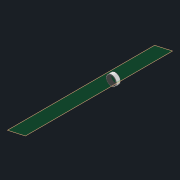
# Autodesk Inventor part: Ball Screw Nut Cap
Saved by Autodesk Inventor 2021 (Build 250183000, 183)
## iProperties
Created: 2020-10-16
Part Number: Ball Screw Nut Cap
Material: Generic
Document SubType Name: Modeling
Designer: Eugene Tang
Density: 1 g/cm^3
Appearance: Default
Mass: 34.4311 g
Surface Area: 123.547 cm^2
Volume: 34.4311 cm^3
Author: Eugene Tang
Autodesk Inventor part; units mm, degrees
ref_plane "YZ Plane" through (0, 0, 0) normal (1, 0, 0) x (0, 1, 0)
ref_plane "XZ Plane" through (0, 0, 0) normal (0, 1, 0) x (-1, 0, 0)
ref_plane "XY Plane" through (0, 0, 0) normal (0, 0, 1) x (1, 0, 0)
sketch "Sketch3" plane through (0, 0, 0) normal (0, 0, 1) x (1, 0, 0)
  circle A0 centre (0.7808, 0) radius 22.0799
  circle A1 centre (0.7808, 0) radius 42.0799
  circle A2 centre (0.7808, 0) radius 18.8799 projected
  dimension "d0" = 44.1598
  dimension "d2" = 20
  constraints: 2 centre point, 1 coincident, 1 concentric
  measures "d0" diameter of A0
  measures "d2" radial gap between concentric circles of A1 A0
extrude "Extrusion1" add sketch "Sketch3" against normal blind 20 contours A1
ref_plane "Work Plane1" through (0.7808, 0, -201) normal (0.2200222, -0.9754949, 0) x (-0.9754949, -0.2200222, 0)
sketch "Sketch5" plane through (0.7808, 0, -201) normal (0.2200222, -0.9754949, 0) x (-0.9754949, -0.2200222, 0)
  line L0 (22.0799, -201) -> (-22.0799, -201) construction
  line L1 (-22.0799, -201) -> (-22.0799, -215.8832) construction
  line L2 (-21.9175, -201) -> (-21.9175, -215.8832) construction
  line L3 (-21.9175, -202.5) -> (-27.3833, -202.5) construction
  line L4 (-23.2165, -201) -> (-23.2165, -206.1611) construction
  line L5 (-23, -201) -> (-23, -205.1917) construction
  line L6 (-26.6968, -201.75) -> (-21.9175, -201.75) construction
  line L7 (-23.2165, -201.75) -> (-21.9175, -201) construction
  line L8 (-23.2165, -201.75) -> (-21.9175, -202.5) construction
  line L9 (-21.9175, -201) -> (-23, -201.625)
  line L10 (-23, -201.625) -> (-23, -201.875)
  line L11 (-23, -201.875) -> (-21.9175, -202.5)
  line L12 (-21.9175, -202.5) -> (-21.9175, -201)
  line L13 (0, -908.6204) -> (0, 268.6204)
  point P0 (0.7616, -201)
  dimension "d16" = 0.1624
  dimension "d17" = 1.5
  dimension "d18" = 1.299
  dimension "d19" = 0.2165
  dimension "d20" = 0.75
  constraints: 26 end point, 9 point on line, 5 vertical, 2 collinear, 1 horizontal, 1 perpendicular, 2 other
  measures "d16" distance between parallel lines of L1 L2
  measures "d17" distance between parallel lines of L3 L0
  measures "d18" distance between parallel lines of L4 L2
  measures "d19" distance between parallel lines of L4 L5
  measures "d20" distance between parallel lines of L3 L6
coil "Coil2" sketch "Sketch5" operation cut axis through (0.7808, 0, 707.6204) along (0, 0, -1) pitch 1.5 turns 13.333333 hand right
sketch "Sketch6" plane through (0.7808, 0, 0) normal (0, 0, 1) x (1, 0, 0)
  circle A0 centre (0, 0) radius 42.0799 construction
  circle A1 centre (0, 0) radius 52.0799
  circle A2 centre (0, 0) radius 32.5
  point P0 (-0.7808, 0)
  dimension "d31" = 65
  dimension "d32" = 10
  constraints: 2 centre point, 2 concentric
  measures "d31" diameter of A2
  measures "d32" radial gap between concentric circles of A0 A1
extrude "Extrusion2" cut sketch "Sketch6" against normal up to surface (20 mm away)
equation "\"d0\" = diameter - 2 * dv + 2 * dvsmall"
equation "\"d3\" = NutCapTread_L"
equation "\"d16\" = 0.125 * dv"
equation "\"d17\" = M20Pitch"
equation "\"d18\" = dv"
equation "\"d19\" = 0.166667 * dv"
equation "\"d20\" = 0.5 * d17"
equation "\"d21\" = M20Pitch"
equation "\"d22\" = NutCapTread_L"
equation "\"d31\" = NutCap_OD"
equation "\"TD\" = 0.5"
equation "\"Ball_DIA\" = 6.35"
equation "\"Screw_L\" = 292"
equation "\"Screw_DIA\" = 36"
equation "\"Nut_OD\" = 66"
equation "\"Flange_DIA\" = 75"
equation "\"Flange_L\" = 5"
equation "\"BPath_REVQ\" = 5.75"
equation "\"Tread_OFFSET\" = 8.405"
equation "\"SteeringColumn_DIA\" = 26"
equation "\"SteeringColumnChamfer_DEG\" = 20deg"
equation "\"Rack_L\" = 307.252"
equation "\"NutCapTread_L\" = 20"
equation "\"NutCapTread_THICKNESS\" = 5"
equation "\"NutCap_THICKNESS\" = 5.38"
equation "\"NutCap_OD\" = 65"
equation "\"diameter\" = 46.32475"
equation "\"dv\" = 1.299"
equation "\"dvsmall\" = 0.2165"
equation "\"M20Pitch\" = 1.5"
body "Solid1"
